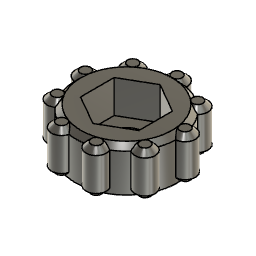
Quarter-20 Knob (Autodesk Fusion 360 design; units mm, degrees)
Autodesk Fusion 360 part; units mm, degrees
sketch "Sketch1" plane through (0, 0, 0) normal (0, 0, 1) x (1, 0, 0) in component "1/4-20 Knob"
  line L0 (-5.75, 3.3198) -> (-5.75, -3.3198)
  line L1 (-5.75, -3.3198) -> (0, -6.6395)
  line L2 (0, -6.6395) -> (5.75, -3.3198)
  line L3 (5.75, -3.3198) -> (5.75, 3.3198)
  line L4 (5.75, 3.3198) -> (0, 6.6395)
  line L5 (0, 6.6395) -> (-5.75, 3.3198)
  circle A0 centre (0, 0) radius 10
  arc A1 (1.99, 9.8) -> (-1.99, 9.8) centre (0, 10) ccw
  circle A2 centre (0, 0) radius 3.5
  dimension "d1" = 11.5
  dimension "d2" = 20
  dimension "d3" = 2
  dimension "d4" = 7
  constraint coincident A0.centre A2.centre
  constraint vertical L0
  constraint coincident A0 A1.start
  constraint coincident A0 A1.end
  constraint coincident A0 A1.centre
  constraint vertical A0.centre A1.centre
  measures "d1" distance of L0 L3
  measures "d2" diameter of A0
  measures "d3" radius of A1
  measures "d4" diameter of A2
extrude "Extrude1" add sketch "Sketch1" against normal blind 2 contours L0 L1 L2 L3 L4 L5 | A0 in component "1/4-20 Knob"
extrude "Extrude2" add sketch "Sketch1" along normal blind 6.5 contours A0 in component "1/4-20 Knob"
extrude "Extrude3" add sketch "Sketch1" along normal blind 6.5 and the other way blind 2 contours A0 A1 in component "1/4-20 Knob"
pattern_circular "C-Pattern2" count 9 over 360 about axis through (0, 0, 1.75) along (0, 0, 1) of "Extrude3" in component "1/4-20 Knob"
chamfer "Chamfer1" distance 1 angle 45 9 edges at (4.1042, -11.2763, -2) (10.3923, -6, -2) (11.8177, 2.0838, -2) (7.7135, 9.1925, -2) (0, 12, -2) (-7.7135, 9.1925, -2) (-11.8177, 2.0838, -2) (-10.3923, -6, -2) (-4.1042, -11.2763, -2) in component "1/4-20 Knob"
chamfer "Chamfer2" distance 1 angle 45 9 edges at (4.1042, -11.2763, 6.5) (-10.3923, -6, 6.5) (-11.8177, 2.0838, 6.5) (-7.7135, 9.1925, 6.5) (0, 12, 6.5) (7.7135, 9.1925, 6.5) (10.3923, -6, 6.5) (-4.1042, -11.2763, 6.5) (11.8177, 2.0838, 6.5) in component "1/4-20 Knob"
chamfer "Chamfer3" distance 1 angle 45 17 edges at (0, -10, 6.5) (-9.8481, -1.7365, 6.5) (-8.6603, 5, 6.5) (-3.4202, 9.3969, 6.5) (3.4202, 9.3969, 6.5) (9.8481, -1.7365, 6.5) (6.4279, -7.6604, 6.5) (-6.4279, -7.6604, 6.5) (9.8481, -1.7365, 6.5) (-9.8481, -1.7365, 6.5) (-3.4202, 9.3969, 6.5) (-6.4279, -7.6604, 6.5) (3.4202, 9.3969, 6.5) (6.4279, -7.6604, 6.5) (-8.6603, 5, 6.5) (0, -10, 6.5) (8.6603, 5, 6.5) in component "1/4-20 Knob"
component "1/4-20 Knob" placed x (1, 0, 0) y (0, 1, 0) z (0, 0, 1) at (0, 0, 0)
